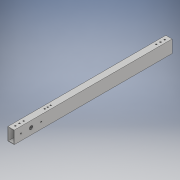
# Autodesk Inventor part: nhk43
Saved by Autodesk Inventor 2019 (Build 230136000, 136)
## iProperties
Created: 2022-02-27
Part Number: nhk43
Material: 一般
Document SubType Name: Sheet Metal
Designer: yuta
Density: 1 g/cm^3
Sheet Metal Rule: Default_mm
Appearance: 既定
Author: yuta
Autodesk Inventor part; units mm, degrees
ref_plane "YZ Plane" through (0, 0, 0) normal (1, 0, 0) x (0, 1, 0)
ref_plane "XZ Plane" through (0, 0, 0) normal (0, 1, 0) x (-1, 0, 0)
ref_plane "XY Plane" through (0, 0, 0) normal (0, 0, 1) x (1, 0, 0)
sketch "スケッチ1" plane through (0, 0, 0) normal (0, 0, 1) x (1, 0, 0)
  line L0 (0, 0) -> (15, 0)
  line L1 (15, 0) -> (15, 30)
  line L2 (15, 30) -> (0, 30)
  line L3 (0, 30) -> (0, 0)
  line L4 (1, 1) -> (14, 1)
  line L5 (14, 1) -> (14, 29)
  line L6 (14, 29) -> (1, 29)
  line L7 (1, 29) -> (1, 1)
  dimension "d0" = 15
  dimension "d1" = 30
  dimension "d2" = 13
  dimension "d3" = 28
  dimension "d4" = 1
  dimension "d5" = 1
  constraints: 16 end point, 4 parallel, 2 horizontal, 2 perpendicular
  measures "d0" distance of L2.end L1.end
  measures "d1" distance of L1.end L0.end
  measures "d2" distance of L6.end L5.end
  measures "d3" distance of L5.end L4.end
  measures "d4" distance between parallel lines of L7 L3
  measures "d5" distance between parallel lines of L0 L4
extrude "押し出し1" add sketch "スケッチ1" along normal blind 375
sketch "スケッチ2" plane through (0, 30, 0) normal (0, 1, 0) x (1, 0, 0)
  circle A0 centre (7.5, -295) radius 1.6
  line L0 (0, 0) -> (0, -375) projected
  line L1 (15, -375) -> (0, -375) projected
  circle A1 centre (7.5, -302) radius 1.6
  circle A2 centre (7.5, -288) radius 1.6
  dimension "d8" = 3.2
  dimension "d9" = 7.5
  dimension "d10" = 80
  dimension "d11" = 3.2
  dimension "d12" = 3.2
  dimension "d13" = 7
  dimension "d14" = 7
  constraints: 3 centre point
  measures "d8" diameter of A0
  measures "d9" distance from line of L0 A0.centre
  measures "d10" distance from line of L1 A0.centre
  measures "d11" diameter of A1
  measures "d12" diameter of A2
  measures "d13" distance of A1.centre A0.centre
  measures "d14" distance of A0.centre A2.centre
hole "穴1" at (7.5, 30, 302) at (7.5, 30, 295) at (7.5, 30, 288) direction (0, -1, 0) diameter 3.2 depth 30
sketch "スケッチ3" plane through (0, 30, 0) normal (0, 1, 0) x (1, 0, 0)
  circle A0 centre (7.5, -10) radius 1.6
  line L0 (15, 0) -> (0, 0) projected
  line L1 (15, 0) -> (15, -375) projected
  circle A1 centre (7.5, -20) radius 1.6
  circle A2 centre (7.5, -30) radius 1.6
  line L2 (15, -187.5) -> (0, -187.5) construction
  line L3 (0, 0) -> (0, -375) projected
  line L4 (15, -375) -> (0, -375) projected
  circle A3 centre (7.5, -365) radius 1.6
  circle A4 centre (7.5, -355) radius 1.6
  circle A5 centre (7.5, -345) radius 1.6
  dimension "d22" = 3.2
  dimension "d23" = 10
  dimension "d24" = 7.5
  dimension "d25" = 3.2
  dimension "d26" = 3.2
  dimension "d27" = 10
  dimension "d28" = 7.5
  dimension "d29" = 10
  dimension "d30" = 7.5
  dimension "d31" = 187.5
  constraints: 6 centre point, 3 symmetric about line, 2 end point, 2 midpoint, 1 horizontal, 3 other
  measures "d22" diameter of A0
  measures "d23" distance from line of L0 A0.centre
  measures "d24" distance from line of L1 A0.centre
  measures "d25" diameter of A1
  measures "d26" diameter of A2
  measures "d27" distance of A1.centre A0.centre
  measures "d28" distance from line of L1 A1.centre
  measures "d29" distance of A1.centre A2.centre
  measures "d30" distance from line of L1 A2.centre
  measures "d31" distance between parallel lines of L4 L2
hole "穴2" at (7.5, 30, 365) at (7.5, 30, 355) at (7.5, 30, 345) at (7.5, 30, 30) at (7.5, 30, 20) at (7.5, 30, 10) direction (0, -1, 0) diameter 3.2 depth 30
sketch "スケッチ4" plane through (0, 30, 0) normal (0, 1, 0) x (1, 0, 0)
  circle A0 centre (7.5, -302) radius 1.6
  line L0 (15, 0) -> (15, -375) projected
  line L1 (15, -375) -> (0, -375) projected
  line L2 (15, 0) -> (15, -375) projected
  line L3 (15, -187.5) -> (0, -187.5) construction
  line L4 (0, 0) -> (0, -375) projected
  dimension "d39" = 3.2
  dimension "d40" = 7.5
  dimension "d41" = 73
  dimension "d42" = 187.5
  constraints: 2 end point, 2 midpoint, 1 centre point, 1 horizontal
  measures "d39" diameter of A0
  measures "d40" distance from line of L0 A0.centre
  measures "d41" distance from line of L1 A0.centre
  measures "d42" distance between parallel lines of L1 L3
extrude "押し出し2" add sketch "スケッチ4" against normal blind 1
sketch "スケッチ5" plane through (0, 0, 0) normal (0, -1, 0) x (1, 0, 0)
  point P0 (0, 0)
sketch "スケッチ6" plane through (0, 0, 0) normal (0, -1, 0) x (1, 0, 0)
  circle A0 centre (7.5, 302) radius 1.6
  line L0 (15, 0) -> (15, 375) projected
  line L1 (0, 375) -> (15, 375) projected
  point P0 (0, 0)
  dimension "d45" = 3.2
  dimension "d46" = 7.5
  dimension "d47" = 73
  constraints: 1 centre point
  measures "d45" diameter of A0
  measures "d46" distance from line of L0 A0.centre
  measures "d47" distance from line of L1 A0.centre
extrude "押し出し3" add sketch "スケッチ6" against normal blind 1
sketch "スケッチ7" plane through (0, 30, 0) normal (0, 1, 0) x (1, 0, 0)
  circle A0 centre (7.5, -281) radius 1.6
  circle A1 centre (7.5, -288) radius 1.6 projected
  line L0 (0, 0) -> (0, -375) projected
  dimension "d50" = 3.2
  dimension "d51" = 7
  dimension "d52" = 7.5
  constraints: 1 centre point
  measures "d50" diameter of A0
  measures "d51" distance of A1.centre A0.centre
  measures "d52" distance from line of L0 A0.centre
extrude "押し出し4" cut sketch "スケッチ7" against normal blind 30 contours A0
sketch "スケッチ8" plane through (15, 0, 0) normal (1, 0, 0) x (0, 0, -1)
  circle A0 centre (-335, 15) radius 4.25
  line L0 (0, 30) -> (-375, 30) projected
  line L1 (-375, 0) -> (-375, 30) projected
  point P0 (0, 0)
  dimension "d55" = 8.5
  dimension "d56" = 15
  dimension "d57" = 40
  constraints: 1 centre point
  measures "d55" diameter of A0
  measures "d56" distance from line of L0 A0.centre
  measures "d57" distance from line of L1 A0.centre
extrude "押し出し5" cut sketch "スケッチ8" against normal blind 30
sketch "スケッチ9" plane through (15, 0, 0) normal (1, 0, 0) x (0, 0, -1)
  circle A0 centre (-359, 15) radius 1.6
  line L0 (0, 30) -> (-375, 30) projected
  line L1 (-375, 0) -> (-375, 30) projected
  line L2 (-335, 0) -> (-335, 30) construction
  circle A1 centre (-311, 15) radius 1.6
  point P0 (0, 0)
  dimension "d60" = 3.2
  dimension "d61" = 15
  dimension "d62" = 16
  dimension "d63" = 40
  constraints: 2 centre point, 2 end point, 1 perpendicular, 1 point on line, 1 symmetric about line, 1 other
  measures "d60" diameter of A0
  measures "d61" distance from line of L0 A0.centre
  measures "d62" distance from line of L1 A0.centre
  measures "d63" distance between parallel lines of L1 L2
hole "穴3" at (15, 15, 359) at (15, 15, 311) direction (-1, 0, 0) diameter 3.2 depth 5
equation "\"BendRadius\" = Thickness"
equation "\"BendReliefWidth\" = Thickness"
equation "\"BendReliefDepth\" = 0.5 * Thickness"
equation "\"CornerReliefSize\" = 4 * Thickness"
equation "\"MinimumRemnant\" = 2 * Thickness"
equation "\"TransitionRadius\" = BendRadius"
equation "\"JacobiRadiusSize\" = BendRadius"
equation "\"GapSize\" = Thickness"
equation "\"Thickness\" = 0.5"
